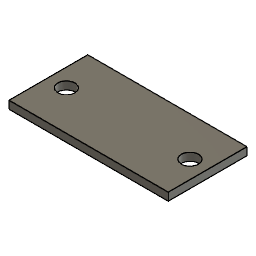
adapter (Autodesk Fusion 360 design; units mm, degrees)
part number: 2026-03-08-16-02-09-308
Autodesk Fusion 360 part; units mm, degrees
sketch "Sketch3" plane through (0, 0, 0) normal (0, 1, 0) x (1, 0, 0)
  line L0 (30.31, 15) -> (-30.31, 15)
  line L1 (-30.31, 15) -> (-30.31, -15)
  line L2 (-30.31, -15) -> (30.31, -15)
  line L3 (30.31, -15) -> (30.31, 15)
  line L4 (30.31, 15) -> (-30.31, -15) construction
  line L5 (-30.31, 15) -> (30.31, -15) construction
  line L6 (-30.31, 0) -> (-23.449, 0)
  circle A0 centre (-23.449, 0) radius 3.25
  line L7 (30.31, 0) -> (23.449, 0)
  circle A1 centre (23.5696, 0) radius 3.25
  dimension "d2" = 60.62
  dimension "d3" = 30
  dimension "d4" = 6.861
  dimension "d5" = 6.5
  dimension "d6" = 6.861
  dimension "d7" = 6.5
  constraint horizontal L0
  constraint perpendicular L0 L1
  constraint parallel L0 L2
  constraint parallel L1 L3
  constraint coincident L4 origin
  constraint coincident L5 origin
  constraint midpoint L1 L6.start
  constraint perpendicular L1 L6
  constraint coincident L6.end A0.centre
  constraint midpoint L3 L7.start
  constraint perpendicular L3 L7
  constraint coincident L7 A1.centre
  measures "d2" distance of L1.end L2.end
  measures "d3" distance of L0.end L1.end
  measures "d4" distance of L6.start L6.end
  measures "d5" diameter of A0
  measures "d6" distance of L7.start L7.end
  measures "d7" diameter of A1
extrude "Extrude1" add sketch "Sketch3" along normal blind 3
